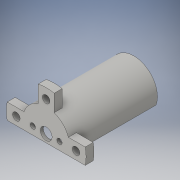
# Autodesk Inventor part: Motor Mount Rack and Pinion
Saved by Autodesk Inventor 2016 (Build 200138000, 138)
## iProperties
Created: 2016-04-18
Part Number: Motor Mount Rack and Pinion
Material: Generic
Document SubType Name: Modeling
Designer: Andrea
Density: 1 g/cm^3
Appearance: Default
Author: Andrea
Autodesk Inventor part; units mm, degrees
ref_plane "YZ Plane" through (0, 0, 0) normal (1, 0, 0) x (0, 1, 0)
ref_plane "XZ Plane" through (0, 0, 0) normal (0, 1, 0) x (-1, 0, 0)
ref_plane "XY Plane" through (0, 0, 0) normal (0, 0, 1) x (1, 0, 0)
sketch "Sketch1" plane through (0, 0, 0) normal (0, 0, 1) x (1, 0, 0)
  arc A0 (14.1527, -5.08) -> (-14.1527, -5.08) centre (0, 0) ccw
  circle A1 centre (0, 0) radius 3.7465
  circle A2 centre (8.509, 0) radius 1.651
  circle A3 centre (-8.509, 0) radius 1.651
  line L0 (-14.1527, -5.08) -> (14.1527, -5.08)
  dimension "d0" = 7.493
  dimension "d1" = 30.0736
  dimension "d2" = 3.302
  dimension "d3" = 8.509
  dimension "d4" = 8.509
  dimension "d7" = 5.08
  constraints: 4 centre point, 2 coincident, 2 end point, 2 horizontal alignment, 2 point on circle, 1 equal radius, 1 horizontal
  measures "d0" diameter of A1
  measures "d1" diameter of A0
  measures "d2" diameter of A2
  measures "d3" distance of A2.centre point (0, 0)
  measures "d4" distance of A3.centre point (0, 0)
  measures "d7" distance from line of L0 A0.centre
extrude "Extrusion1" add sketch "Sketch1" along normal blind 1.905
sketch "Sketch3" plane through (0, 0, 0) normal (0, 0, -1) x (-1, 0, 0)
  arc A0 (14.1527, -5.08) -> (-14.1527, -5.08) centre (0, 0) ccw
  arc A1 (11.4177, -5.08) -> (-11.4177, -5.08) centre (0, 0) ccw
  line L0 (-14.1527, -5.08) -> (14.1527, -5.08)
  dimension "d8" = 30.0736
  dimension "d9" = 24.9936
  dimension "d10" = 5.08
  constraints: 4 point on circle, 2 centre point, 2 coincident, 2 end point, 2 point on line, 1 horizontal
  measures "d8" diameter of A0
  measures "d9" diameter of A1
  measures "d10" distance from line of point (0, 0) L0
extrude "Extrusion2" add sketch "Sketch3" along normal blind 53.975 contours L0 A1 A0
sketch "Sketch4" plane through (0, 0, 1.905) normal (0, 0, 1) x (1, 0, 0)
  arc A0 (14.1527, -5.08) -> (-14.1527, -5.08) centre (0, 0) ccw projected
  arc A1 (14.1527, -5.08) -> (-14.1527, -5.08) centre (0, 0) ccw
  line L0 (-14.1527, -5.08) -> (14.1527, -5.08) projected
  line L1 (-5.08, 24.8868) -> (-5.08, 14.1527)
  line L2 (5.08, 24.8868) -> (5.08, 14.1527)
  arc A2 (-24.8868, 5.08) -> (-24.8868, -5.08) centre (0, 0) ccw
  arc A3 (24.8868, -5.08) -> (24.8868, 5.08) centre (0, 0) ccw
  arc A4 (5.08, 24.8868) -> (-5.08, 24.8868) centre (0, 0) ccw
  line L3 (-24.8868, 5.08) -> (-14.1527, 5.08)
  line L4 (14.1527, 5.08) -> (24.8868, 5.08)
  line L5 (-24.8868, -5.08) -> (-14.1527, -5.08)
  line L6 (14.1527, -5.08) -> (24.8868, -5.08)
  dimension "d14" = 30.0736
  dimension "d20" = 5.08
  dimension "d21" = 5.08
  dimension "d22" = 25.4
  dimension "d23" = 25.4
  dimension "d24" = 25.4
  dimension "d25" = 10.16
  dimension "d27" = 10.16
  constraints: 14 end point, 14 point on circle, 4 centre point, 4 horizontal, 2 coincident, 2 collinear, 2 vertical
  measures "d14" diameter of A1
  measures "d20" distance from line of L2 point (0, 0)
  measures "d21" horizontal distance of L1.start point (0, 0)
  measures "d22" radius of A4
  measures "d23" radius of A3
  measures "d24" radius of A2
  measures "d25" distance between parallel lines of L0 L4
  measures "d27" distance between parallel lines of L0 L3
extrude "Extrusion3" add sketch "Sketch4" against normal blind 5.08 contours A0 L4 A3 L6 | L5 A2 L3 A0 | A0 L1 A4 L2
sketch "Sketch5" plane through (0, 0, 1.905) normal (0, 0, 1) x (1, 0, 0)
  circle A0 centre (-19.05, 0) radius 2.3813
  circle A1 centre (19.05, 0) radius 2.3813
  circle A2 centre (0, 19.05) radius 2.3813
  point P0 (0, 0)
  dimension "d31" = 4.7625
  dimension "d32" = 19.05
  dimension "d33" = 19.05
  dimension "d34" = 19.05
  constraints: 3 centre point, 2 equal radius, 2 horizontal alignment, 1 vertical alignment
  measures "d31" diameter of A0
  measures "d32" distance of A0.centre point (0, 0)
  measures "d33" distance of A1.centre point (0, 0)
  measures "d34" distance of A2.centre point (0, 0)
extrude "Extrusion4" cut sketch "Sketch5" against normal up to surface (5.08 mm away)
equation "\"d4\" = d3"
equation "\"d21\" = d20"
equation "\"d22\" = d23"
equation "\"d24\" = d23"
equation "\"d27\" = d25"
equation "\"d33\" = d32"
equation "\"d34\" = d32"
body "Solid1"
